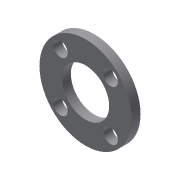
# Autodesk Inventor part: BarrelHubAdapter
Saved by Autodesk Inventor 2018 (Build 220112000, 112)
## iProperties
Created: 2019-04-12
Part Number: BarrelHubAdapter
Material: Generic
Document SubType Name: Modeling
Designer: ball
Density: 1 g/cm^3
Appearance: Default
Author: ball
Autodesk Inventor part; units mm, degrees
ref_plane "YZ Plane" through (0, 0, 0) normal (1, 0, 0) x (0, 1, 0)
ref_plane "XZ Plane" through (0, 0, 0) normal (0, 1, 0) x (-1, 0, 0)
ref_plane "XY Plane" through (0, 0, 0) normal (0, 0, 1) x (1, 0, 0)
sketch "Sketch1" plane through (0, 0, 0) normal (0, 0, 1) x (1, 0, 0)
  circle A0 centre (0, 0) radius 6.35 construction
  spline S0 degree 3 number of poles 388 construction
  spline S1 degree 3 number of poles 388 construction
  spline S2 degree 3 number of poles 388 construction
  spline S3 degree 3 number of poles 388 construction
  arc A1 (-3.2013, -9.3003) -> (3.2013, -9.3003) centre (0, 0) ccw construction
  arc A2 (3.2013, 9.3003) -> (-3.2013, 9.3003) centre (0, 0) ccw construction
  circle A3 centre (0, 0) radius 6.477
  circle A4 centre (0, 0) radius 12.7
  arc A5 (8.4339, 6.0408) -> (7.3595, 5.2195) centre (6.9148, 6.9148) ccw construction
  arc A6 (6.0408, -8.4339) -> (5.2195, -7.3595) centre (6.9148, -6.9148) ccw construction
  arc A7 (-6.0408, 8.4339) -> (-5.2195, 7.3595) centre (-6.9148, 6.9148) ccw construction
  arc A8 (-8.4339, -6.0408) -> (-7.3595, -5.2195) centre (-6.9148, -6.9148) ccw construction
  circle A9 centre (6.9148, 6.9148) radius 1.9685
  circle A10 centre (6.9148, -6.9148) radius 1.9685
  circle A11 centre (-6.9148, 6.9148) radius 1.9685
  circle A12 centre (-6.9148, -6.9148) radius 1.9685
  dimension "d0" = 12.954
  dimension "d1" = 25.4
  dimension "d2" = 3.937
  dimension "d3" = 3.937
  dimension "d4" = 3.937
  dimension "d5" = 3.937
  constraints: 9 centre point, 6 coincident, 4 point on circle, 26 other
  measures "d0" diameter of A3
  measures "d1" diameter of A4
  measures "d2" diameter of A9
  measures "d3" diameter of A10
  measures "d4" diameter of A11
  measures "d5" diameter of A12
extrude "Extrusion1" add sketch "Sketch1" along normal blind 2.413
body "Solid1"
